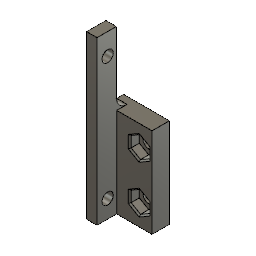
Alu_Mount_Adapter (Autodesk Fusion 360 design; units mm, degrees)
Autodesk Fusion 360 part; units mm, degrees
sketch "Sketch1" plane through (231.1286, 0, 0) normal (-1, 0, 0) x (0, 0, 1)
  circle A0 centre (423.85, -235.9668) radius 1.5
  circle A1 centre (423.85, -270.828) radius 1.5
  line L0 (421.35, -229.9414) -> (421.35, -275.9414)
  line L1 (421.35, -275.9414) -> (426.85, -275.9414)
  line L2 (426.85, -275.9414) -> (426.85, -229.9414)
  line L3 (426.85, -229.9414) -> (421.35, -229.9414)
  circle A2 centre (423.85, -235.9668) radius 4
  dimension "d22" = 8
  measures "d22" diameter of A2
extrude "Extrude1" add sketch "Sketch1" along normal blind 4 contours L0 L2 L3 A2 | L0 L2 A2 | L0 L1 L2 A2
sketch "Sketch2" plane through (0, 0, 421.35) normal (0, 0, -1) x (-1, 0, 0)
  line L0 (-231.1286, -229.9414) -> (-231.1286, -275.9414)
  line L1 (-231.1286, -275.9414) -> (-227.1286, -275.9414)
  line L2 (-227.1286, -275.9414) -> (-227.1286, -229.9414)
  line L3 (-227.1286, -229.9414) -> (-231.1286, -229.9414)
  line L4 (-233.6257, -250.5312) -> (-240.5303, -250.5312)
  line L5 (-233.6257, -275.9414) -> (-240.6765, -275.9414)
  line L6 (-231.1286, -275.9414) -> (-227.1286, -275.9414)
  line L7 (-227.1286, -275.9414) -> (-227.1286, -250.5312)
  line L8 (-227.1286, -250.5312) -> (-231.1286, -250.5312)
  line L9 (-231.1286, -250.5312) -> (-231.1286, -275.9414)
extrude "Extrude2" add sketch "Sketch2" along normal blind 5 contours L0 L1 L2 L6 L7 L8 L9
sketch "Sketch3" plane through (231.1286, 0, 0) normal (1, 0, 0) x (0, 0, -1)
  circle A0 centre (-423.85, -235.9668) radius 1.5
  circle A1 centre (-423.85, -270.828) radius 1.5
  line L0 (-421.35, -229.9414) -> (-426.85, -229.9414)
  line L1 (-426.85, -229.9414) -> (-426.85, -275.9414)
  line L2 (-426.85, -275.9414) -> (-416.35, -275.9414)
  line L3 (-416.35, -275.9414) -> (-416.35, -250.5312)
  line L4 (-416.35, -250.5312) -> (-421.35, -250.5312)
  line L5 (-421.35, -250.5312) -> (-421.35, -229.9414)
  line L6 (-421.35, -275.9414) -> (-421.35, -229.9414)
extrude "Extrude3" add sketch "Sketch3" along normal blind 10 contours L2 L3 L4 L6
fillet "Fillet1" radius 3 1 edges at (229.1286, -250.5312, 421.35)
sketch "Sketch4" plane through (0, 0, 421.35) normal (0, 0, 1) x (1, 0, 0)
  line L0 (231.1286, -250.5312) -> (231.1286, -275.9414)
  line L1 (231.1286, -275.9414) -> (241.1286, -275.9414)
  line L2 (241.1286, -275.9414) -> (241.1286, -250.5312)
  line L3 (241.1286, -250.5312) -> (231.1286, -250.5312)
  circle A0 centre (237.4786, -256.5312) radius 1.6
  circle A1 centre (237.4786, -269.9414) radius 1.6
hole "Hole1" at (237.4786, -269.9414, 421.35) at (237.4786, -256.5312, 421.35) direction (0, 0, -1) diameter 3.2 depth 5 tip angle 180
move_face "OffsetFaces1" offset -0.1 1 faces at (228.462, -271.3411, 425.2595)
move_face "OffsetFaces2" offset -0.1 1 faces at (228.462, -234.893, 422.8026)
move_face "OffsetFaces3" offset -0.05 1 faces at (232.7488, -265.2765, 421.35)
move_face "OffsetFaces4" offset -1 1 faces at (227.1286, -265.5355, 418.3695)
sketch "Sketch5" plane through (0, 0, 421.3) normal (0, 0, 1) x (1, 0, 0)
  circle A0 centre (237.4786, -269.9414) radius 1.6
  circle A1 centre (237.4786, -256.5312) radius 1.6
  line L0 (231.1286, -250.5312) -> (231.1286, -275.9414)
  line L1 (231.1286, -275.9414) -> (241.1286, -275.9414)
  line L2 (241.1286, -275.9414) -> (241.1286, -250.5312)
  line L3 (241.1286, -250.5312) -> (231.1286, -250.5312)
  circle A2 centre (237.4786, -256.5312) radius 1.6
  circle A3 centre (237.4786, -269.9414) radius 1.6
  line L4 (237.4786, -256.5312) -> (237.4786, -269.9414) construction
  line L5 (237.4786, -259.5912) -> (240.1287, -258.0612)
  line L6 (240.1287, -258.0612) -> (240.1287, -255.0012)
  line L7 (240.1287, -255.0012) -> (237.4786, -253.4712)
  line L8 (237.4786, -253.4712) -> (234.8286, -255.0012)
  line L9 (234.8286, -255.0012) -> (234.8286, -258.0612)
  line L10 (234.8286, -258.0612) -> (237.4786, -259.5912)
  line L11 (237.4786, -266.8814) -> (234.8286, -268.4114)
  line L12 (234.8286, -268.4114) -> (234.8286, -271.4714)
  line L13 (234.8286, -271.4714) -> (237.4786, -273.0014)
  line L14 (237.4786, -273.0014) -> (240.1287, -271.4714)
  line L15 (240.1287, -271.4714) -> (240.1287, -268.4114)
  line L16 (240.1287, -268.4114) -> (237.4786, -266.8814)
  dimension "d37" = 3.06
  dimension "d38" = 3.06
extrude "Extrude4" cut sketch "Sketch5" against normal blind 2.7 contours L5 L6 L7 L8 L9 L10 | L11 L12 L13 L14 L15 L16
chamfer "Chamfer1" distance 0.4 angle 45 12 edges at (234.8286, -256.5312, 421.3) (236.1536, -254.2362, 421.3) (238.8037, -254.2362, 421.3) (240.1287, -256.5312, 421.3) (238.8037, -258.8262, 421.3) (236.1536, -258.8262, 421.3) (236.1536, -267.6464, 421.3) (234.8286, -269.9414, 421.3) (236.1536, -272.2364, 421.3) (238.8037, -272.2364, 421.3) (240.1287, -269.9414, 421.3) (238.8037, -267.6464, 421.3)
